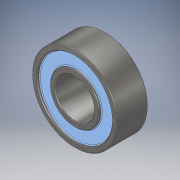
# Autodesk Inventor part: MR115 2RS
Saved by Autodesk Inventor 2019 (Build 230136000, 136)
## iProperties
Created: 2018-10-20
Part Number: MR115 2RS
Material: Steel, Alloy
Document SubType Name: Modeling
Designer: LillaHunden
Density: 7.73 g/cm^3
Appearance: Semi-Polished
Author: LillaHunden
Autodesk Inventor part; units mm, degrees
ref_plane "YZ Plane" through (0, 0, 0) normal (1, 0, 0) x (0, 1, 0)
ref_plane "XZ Plane" through (0, 0, 0) normal (0, 1, 0) x (-1, 0, 0)
ref_plane "XY Plane" through (0, 0, 0) normal (0, 0, 1) x (1, 0, 0)
sketch "Sketch1" plane through (0, 0, 0) normal (0, 0, 1) x (1, 0, 0)
  circle A0 centre (0, 0) radius 5.5
  dimension "d0" = 11
  constraints: 1 centre point, 1 coincident
  measures "d0" diameter of A0
extrude "Extrusion1" add sketch "Sketch1" along normal blind 4
sketch "Sketch2" plane through (0, 0, 4) normal (0, 0, 1) x (1, 0, 0)
  circle A0 centre (0, 0) radius 2.5
  dimension "d3" = 5
  constraints: 1 centre point, 1 coincident
  measures "d3" diameter of A0
extrude "Extrusion2" cut sketch "Sketch2" against normal through all
sketch "Sketch3" plane through (0, 0, 4) normal (0, 0, 1) x (1, 0, 0)
  circle A0 centre (0, 0) radius 3.2
  circle A1 centre (0, 0) radius 4.8
  circle A2 centre (0, 0) radius 2.5 projected
  circle A3 centre (0, 0) radius 5.5 projected
  dimension "d6" = 0.7
  dimension "d7" = 0.7
  constraints: 2 centre point, 2 coincident
  measures "d6" radial gap between concentric circles of A0 A2
  measures "d7" radial gap between concentric circles of A3 A1
extrude "Extrusion3" cut sketch "Sketch3" against normal blind 0.3 contours A1
chamfer "Chamfer1" distance 0.1 angle 45 4 edges at (-4.8, 0, 4) (-5.5, 0, 4) (-3.2, 0, 4) (-2.5, 0, 4)
fillet "Fillet1" radius 0.1 2 edges at (-4.8, 0, 3.7) (-3.2, 0, 3.7)
ref_plane "Work Plane1" through (0, 0, 2) normal (0, 0, 1) x (1, 0, 0)
mirror "Mirror1" about plane through (0, 0, 2) normal (0, 0, 1) of "Extrusion3", "Fillet1"
chamfer "Chamfer2" distance 0.1 angle 45 3 edges at (-5.5, 0, 0) (-4.8, 0, 0) (-2.5, 0, 0)
body "Solid1"
